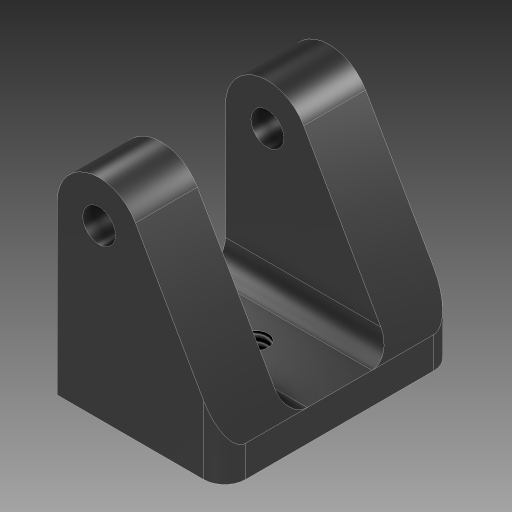
# Autodesk Inventor part: Cascade Pulley Block2 (WCP-0298)
Saved by Autodesk Inventor 2024 (Build 280153000, 153)
## iProperties
Created: 2023-03-23
Part Number: Cascade Pulley Block2 (WCP-0298)
Material: Aluminum 6061
Document SubType Name: Modeling
Designer: Max Boord
Density: 2.7 g/cm^3
Appearance: Glossy - Black
Mass: 33.1065 g
Surface Area: 55.6629 cm^2
Volume: 12.2617 cm^3
Author: Max Boord
Autodesk Inventor part; units mm, degrees
ref_plane "YZ Plane" through (0, 0, 0) normal (1, 0, 0) x (0, 1, 0)
ref_plane "XZ Plane" through (0, 0, 0) normal (0, 1, 0) x (-1, 0, 0)
ref_plane "XY Plane" through (0, 0, 0) normal (0, 0, 1) x (1, 0, 0)
sketch "Sketch1" plane through (0, 0, 0) normal (0, 0, 1) x (1, 0, 0)
  line L0 (-12.7, 0) -> (12.7, 0)
  line L1 (12.7, 0) -> (12.7, 4.7625)
  line L2 (12.7, 4.7625) -> (-0.831, 28.5406)
  line L3 (-12.7, 25.4) -> (-12.7, 0)
  arc A0 (-0.831, 28.5406) -> (-12.7, 25.4) centre (-6.35, 25.4) ccw
  circle A1 centre (-6.35, 25.4) radius 2.4892
  point P0 (0, 0)
  point P1 (0, 0)
  dimension "d0" = 25.4
  dimension "d1" = 6.35
  dimension "d2" = 4.7625
  dimension "d3" = 25.4
  dimension "d4" = 4.9784
  constraints: 8 end point, 2 centre point, 2 coincident, 2 point on circle, 2 tangent, 1 horizontal, 1 midpoint, 1 perpendicular, 1 vertical
  measures "d0" distance of L0.start L0.end
  measures "d1" radius of A0
  measures "d2" distance of L0.end L1.end
  measures "d3" distance from line of L0 A0.centre
  measures "d4" diameter of A1
extrude "Extrusion1" add sketch "Sketch1" along normal mid plane 34.925
sketch "Sketch2" plane through (12.7, 0, 17.4625) normal (1, 0, 0) x (0, 0, -1)
  line L0 (34.925, 4.7625) -> (0, 4.7625) projected
  line L1 (9.398, 31.75) -> (9.398, 7.9375)
  line L2 (12.573, 4.7625) -> (22.352, 4.7625)
  line L3 (25.527, 7.9375) -> (25.527, 31.75)
  arc A0 (9.398, 7.9375) -> (12.573, 4.7625) centre (12.573, 7.9375) ccw
  arc A1 (22.352, 4.7625) -> (25.527, 7.9375) centre (22.352, 7.9375) ccw
  line L4 (0, 0) -> (34.925, 0) construction
  line L5 (34.925, 31.75) -> (0, 31.75) projected
  point P0 (17.4625, 0)
  point P1 (17.4625, 4.7625)
  point P2 (17.4625, 0)
  point P3 (12.573, 4.7625)
  point P4 (22.352, 4.7625)
  dimension "d7" = 3.175
  dimension "d8" = 16.129
  constraints: 6 end point, 4 point on circle, 4 tangent, 2 centre point, 2 midpoint, 2 perpendicular, 2 point on line, 1 collinear, 1 equal radius, 1 vertical, 1 vertical alignment
  measures "d7" radius of A0
  measures "d8" distance between parallel lines of L3 L1
extrude "Extrusion2" cut sketch "Sketch2" against normal through all
chamfer "Chamfer2" [suppressed]
chamfer "Chamfer3" [suppressed]
fillet "Fillet1" radius 3.175 2 edges at (12.7, 2.3813, 17.4625) (12.7, 2.3813, -17.4625)
sketch "Sketch3" plane through (-12.7, 0, -17.4625) normal (0, -1, 0) x (1, 0, 0)
  line L0 (12.7, 30.1625) -> (12.7, 4.7625) construction
  point P0 (12.7, 17.4625)
  point P1 (12.7, 17.4625)
  point P2 (12.7, 17.4625)
  dimension "d12" = 25.4
  dimension "d37" = 38.1
  dimension "d38" = 25.4
  dimension "d32" = 25.4
  dimension "d33" = 25.4
  dimension "d34" = 50.8
  constraints: 3 coincident, 2 end point, 1 midpoint, 1 vertical
  measures "d12" distance of L0.start L0.end
hole "Hole1" at (0, 0, -12.7) at (0, 0, 12.7) at (0, 0, 0) direction (0, 1, 0) diameter 3.683 depth 19.05 tip angle 118 thread size "10-24 UNC" class "2B" standard "ANSI Unified Screw Threads"
pattern_linear "Rectangular Pattern1" [suppressed]
equation "\"d32\" = d33"
body "Solid1"
